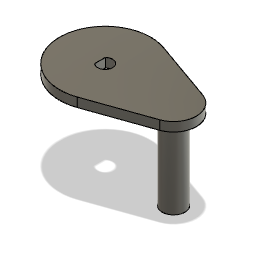
3.DriverWheel (Autodesk Fusion 360 design; units mm, degrees)
Autodesk Fusion 360 part; units mm, degrees
sketch "Sketch1" plane through (0, 0, 0) normal (0, 1, 0) x (1, 0, 0)
  circle A0 centre (30, 0) radius 5
  line L0 (33.328, 9.43) -> (6.6508, 18.845)
  line L1 (33.328, -9.43) -> (6.6508, -18.845)
  arc A1 (33.328, -9.43) -> (33.328, 9.43) centre (30, 0) ccw
  arc A2 (6.6508, 18.845) -> (6.6508, -18.845) centre (0, 0) ccw
  line L2 (-2.25, 2.3452) -> (-2.25, -2.3452)
  arc A3 (-2.25, -2.3452) -> (-2.25, 2.3452) centre (0, 0) ccw
  constraint coincident A2.centre A3.centre
  constraint concentric A0 A1
  constraint tangent L0 A2
  constraint tangent L0 A1
  constraint concentric A2 A3
extrude "Extrude1" add sketch "Sketch1" along normal blind 4 contours A0 | L0 L1 A1 A2
extrude "Extrude2" add sketch "Sketch1" against normal blind 35 contours A0
